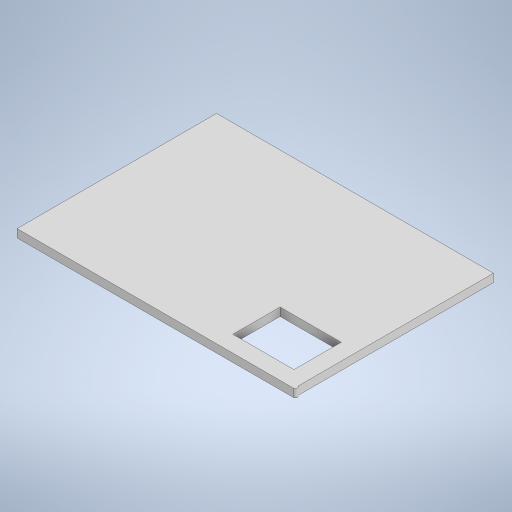
# Autodesk Inventor part: side_lid_yes_hole
Saved by Autodesk Inventor 2023 (Build 270158000, 158)
## iProperties
Created: 2023-05-26
Part Number: side_lid_yes_hole
Material: Generic
Document SubType Name: Modeling
Designer: jxl19
Density: 1 g/cm^3
Appearance: Default
Author: jxl19
## iProperties of the stored document side_lid_yes_hole_3DPrint.ipt
Created: 2023-05-26
Part Number: side_lid_yes_hole_3DPrint
Material: Generic
Document SubType Name: Modeling
Designer: jxl19
Density: 1 g/cm^3
Appearance: Default
Author: jxl19
Autodesk Inventor part; units mm, degrees
ref_plane "YZ Plane" through (0, 0, 0) normal (1, 0, 0) x (0, 1, 0)
ref_plane "XZ Plane" through (0, 0, 0) normal (0, 1, 0) x (-1, 0, 0)
ref_plane "XY Plane" through (0, 0, 0) normal (0, 0, 1) x (1, 0, 0)
sketch "Sketch1" plane through (0, 0, 0) normal (0, 1, 0) x (-1, 0, 0)
  line L0 (-34, 24.5) -> (34, 24.5)
  line L1 (34, 24.5) -> (34, -24.5)
  line L2 (34, -24.5) -> (-34, -24.5)
  line L3 (-34, -24.5) -> (-34, 24.5)
  line L4 (-34, 24.5) -> (34, -24.5) construction
  line L5 (34, 24.5) -> (-34, -24.5) construction
  point P0 (0, 0)
  dimension "d0" = 49
  dimension "d1" = 68
  constraints: 12 end point, 2 midpoint, 2 parallel, 1 horizontal, 1 perpendicular
  measures "d0" distance of L0.end L1.end
  measures "d1" distance of L1.end L2.end
extrude "Extrusion1" add sketch "Sketch1" along normal blind 2
sketch "Sketch3" plane through (0, 2, 0) normal (0, 1, 0) x (1, 0, 0)
  line L0 (-34, -24.5) -> (34, -24.5) projected
  line L1 (34, -24.5) -> (34, 24.5) projected
  arc A0 (34, -24.5) -> (34, -23.5) centre (33.818, -24) ccw
  point P0 (0, 0)
  dimension "d6" = 1
  dimension "d9" = 140
  constraints: 2 point on circle, 1 centre point, 1 point on line
  measures "d6" distance of L0.end A0.end
extrude "Extrusion2" add sketch "Sketch3" against normal blind 2
sketch "Sketch4" plane through (0, 2, 0) normal (0, 1, 0) x (1, 0, 0)
  line L0 (15, -8.9) -> (30, -8.9)
  line L1 (30, -8.9) -> (30, -20.5)
  line L2 (30, -20.5) -> (15, -20.5)
  line L3 (15, -20.5) -> (15, -8.9)
  line L4 (15, -8.9) -> (30, -20.5) construction
  line L5 (30, -8.9) -> (15, -20.5) construction
  line L6 (34, -23.5) -> (34, 24.5) projected
  line L7 (-34, -24.5) -> (34, -24.5) projected
  point P0 (0, 0)
  point P1 (22.5, -14.7)
  dimension "d12" = 15
  dimension "d13" = 11.6
  dimension "d14" = 4
  dimension "d15" = 4
  constraints: 12 end point, 2 midpoint, 2 parallel, 1 horizontal, 1 perpendicular
  measures "d12" distance of L0.start L0.end
  measures "d13" distance of L0.end L1.end
  measures "d14" distance between parallel lines of L6 L1
  measures "d15" distance between parallel lines of L7 L2
extrude "Extrusion3" cut sketch "Sketch4" against normal blind 10
body "Solid1"
